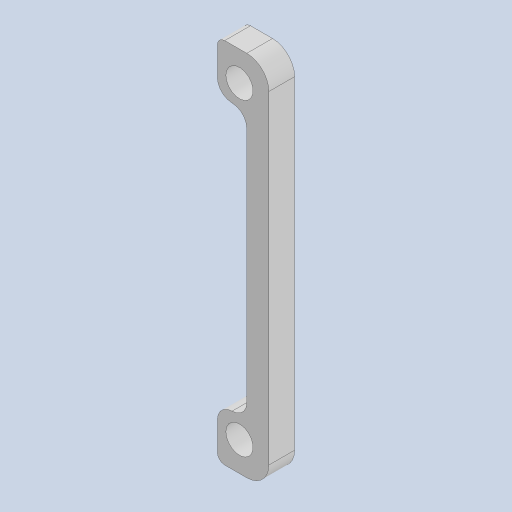
# Autodesk Inventor part: door_center_03
Saved by Autodesk Inventor 2024.4 (Build 284460030, 460C)
## iProperties
Created: 2026-07-13
Part Number: door_center_03
Material: Generic
Document SubType Name: Modeling
Designer: tooles01
Density: 1 g/cm^3
Appearance: Default
Author: tooles01
Autodesk Inventor part; units mm, degrees
ref_plane "YZ Plane" through (0, 0, 0) normal (1, 0, 0) x (0, 1, 0)
ref_plane "XZ Plane" through (0, 0, 0) normal (0, 1, 0) x (-1, 0, 0)
ref_plane "XY Plane" through (0, 0, 0) normal (0, 0, 1) x (1, 0, 0)
derived "door_front_04.ipt"
sketch "Sketch1: base" plane through (0, 0, 0) normal (0, 0, 1) x (1, 0, 0)
  line L0 (-41, 50) -> (23, 50)
  line L1 (23, 50) -> (23, 0)
  line L2 (23, 0) -> (-41, 0)
  line L3 (-41, 0) -> (-41, 50)
  circle A0 centre (0, 30) radius 16.25
  line L4 (-37, 46) -> (19, 46) construction
  line L5 (19, 46) -> (19, 4) construction
  line L6 (19, 4) -> (-37, 4) construction
  line L7 (-37, 4) -> (-37, 46) construction
  point P0 (0, 0)
sketch "Sketch: base" plane through (0, 0, 0) normal (0, 0, 1) x (1, 0, 0)
  line L0 (-41, 50) -> (23, 50) projected
  line L1 (-41, 0) -> (-41, 50) projected
  line L2 (23, 50) -> (23, 0) projected
  line L3 (-41, 42) -> (23, 42) construction
  circle A0 centre (-37, 46) radius 1.85 construction
  line L4 (23, 0) -> (-41, 0) projected
  circle A1 centre (0, 30) radius 16.25 construction
  line L5 (16, 50) -> (16, 0)
  circle A2 centre (19, 46) radius 1.85 construction
  line L6 (16, 43.15) -> (20, 43.15)
  line L7 (20, 43.15) -> (20, 6.85)
  line L8 (20, 6.85) -> (16, 6.85)
  point P0 (0, 0)
  point P1 (19, 4)
  point P2 (16, 42)
  point P3 (20, 42)
  dimension "d15" = 8
  dimension "d36" = 3.7
  dimension "d51" = 7
  dimension "sk_M3_through_hole" = 3.7
  dimension "d54" = 2.85
  dimension "d56" = 4
  dimension "d57" = 2.85
  constraints: 10 end point, 6 point on line, 5 perpendicular, 2 centre point, 2 coincident
  measures "d15" distance between parallel lines of L0 L3
  measures "d36" diameter of A0
  measures "d51" distance between parallel lines of L2 L5
  measures "sk_M3_through_hole" diameter of A2
  measures "d54" distance from line of L6 point (19, 46)
  measures "d56" distance of L6.start L6.end
  measures "d57" distance from line of point (19, 4) L8
sketch "Sketch: text" plane through (0, 0, 0) normal (0, 0, 1) x (1, 0, 0)
  line L0 (9.5, 47.5) -> (12.5, 47.5) construction
  line L1 (12.5, 47.5) -> (12.5, 44.5) construction
  line L2 (12.5, 44.5) -> (9.5, 44.5) construction
  line L3 (9.5, 44.5) -> (9.5, 47.5) construction
  line L4 (-41, 50) -> (23, 50) construction
  line L5 (-41, 42) -> (23, 42) construction
  line L6 (23, 50) -> (23, 42) construction
  point P0 (0, 0)
  point P1 (11, 47.5)
  point P2 (-9, 50)
  point P3 (9.5, 46)
  point P4 (12.5, 46)
  point P5 (23, 46)
  dimension "d12" = 3
  dimension "d16" = 12
  constraints: 5 midpoint, 2 end point, 1 horizontal, 1 horizontal alignment, 1 perpendicular, 2 other
  measures "d12" distance of L0.start L0.end
  measures "d16" distance from line of L6 point (11, 47.5)
extrude "Ex1: base" add sketch "Sketch: base" against normal blind 3.5 contours L0 L2 L4 L5 L8 L7 L6
extrude "Ex2: text" [suppressed]
hole "Hole1: mounting (M3 thru holes)" at (19, 46, 0) at (-37, 46, 0) at (19, 4, 0) direction (0, 0, -1) diameter 3.7 end through all both
fillet "Fillet1" radius 3 2 edges at (23, 50, -1.75) (23, 0, -1.75)
fillet "Fillet2" radius 2 4 edges at (20, 43.15, -1.75) (20, 6.85, -1.75) (16, 6.85, -1.75) (16, 43.15, -1.75)
fillet "Fillet3" radius 1 2 edges at (16, 50, -1.75) (16, 0, -1.75)
equation "\"sk_M3_through_hole\" = M3_through_hole"
equation "\"d57\" = d54"
equation "\"d61\" = 4.2"
equation "\"M3_through_hole\" = 3.7"
body "Solid1"
